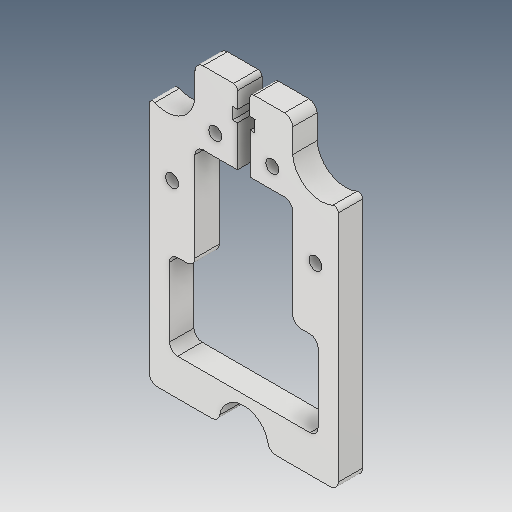
# Autodesk Inventor part: Hotend Slide Part 2
Saved by Autodesk Inventor 2017 (Build 210142000, 142)
## iProperties
Created: 2016-06-24
Part Number: Hotend Slide Part 2
Material: Acetal Resin, White
Document SubType Name: Modeling
Designer: joshm
Density: 1.425 g/cm^3
Appearance: Smooth - White
Mass: 13.5596 g
Surface Area: 60.0881 cm^2
Volume: 9.51552 cm^3
Author: joshm
Autodesk Inventor part; units mm, degrees
ref_plane "YZ Plane" through (0, 0, 0) normal (1, 0, 0) x (0, 1, 0)
ref_plane "XZ Plane" through (0, 0, 0) normal (0, 1, 0) x (-1, 0, 0)
ref_plane "XY Plane" through (0, 0, 0) normal (0, 0, 1) x (1, 0, 0)
sketch "Sketch1" plane through (0, 0, 0) normal (0, 0, 1) x (1, 0, 0)
  line L0 (-11.9794, 21.8002) -> (-11.9794, -0.1998)
  line L1 (-13.9794, -2.1998) -> (-16.2294, -2.1998)
  line L2 (12.0206, -0.1998) -> (12.0206, 21.8002)
  line L3 (16.2706, -2.1998) -> (14.0206, -2.1998)
  line L4 (-23.2294, -2.1998) -> (-23.2294, 27.0455)
  line L5 (23.2706, -2.1998) -> (23.2706, 27.0455)
  line L6 (-1.5294, 33.8002) -> (-2.7294, 33.8002)
  line L7 (1.5706, 33.8002) -> (2.7706, 33.8002)
  arc A0 (12.0206, 33.8002) -> (21.8617, 27.958) centre (18.9993, 34.346) ccw
  arc A1 (-21.8205, 27.958) -> (-11.9794, 33.8002) centre (-18.9581, 34.346) ccw
  line L8 (-1.5294, 23.8002) -> (-1.5294, 33.8002)
  line L9 (1.5706, 23.8002) -> (1.5706, 33.8002)
  circle A2 centre (17.6456, 13.5013) radius 1.6
  circle A3 centre (-17.6044, 13.5013) radius 1.6
  circle A4 centre (7.0206, 28.8002) radius 1.6
  circle A5 centre (-6.9794, 28.8002) radius 1.6
  line L10 (-1.5294, 33.8002) -> (-2.7294, 33.8002)
  line L11 (2.7706, 33.8002) -> (2.7706, 36.7002)
  line L12 (-2.7294, 36.7002) -> (-2.7294, 33.8002)
  line L13 (-2.4794, 41.7002) -> (-9.9794, 41.7002)
  line L14 (-11.9794, 39.7002) -> (-11.9794, 33.8002)
  line L15 (12.0206, 33.8002) -> (12.0206, 39.7002)
  line L16 (10.0206, 41.7002) -> (2.5206, 41.7002)
  line L17 (1.5206, 36.7002) -> (1.5206, 40.7002)
  line L18 (-1.4794, 40.7002) -> (-1.4794, 36.7002)
  arc A6 (-9.9794, 23.8002) -> (-11.9794, 21.8002) centre (-9.9794, 21.8002) ccw
  arc A7 (12.0206, 21.8002) -> (10.0206, 23.8002) centre (10.0206, 21.8002) ccw
  arc A8 (12.0206, -0.1998) -> (14.0206, -2.1998) centre (14.0206, -0.1998) ccw
  arc A9 (-13.9794, -2.1998) -> (-11.9794, -0.1998) centre (-13.9794, -0.1998) ccw
  arc A10 (12.0206, 39.7002) -> (10.0206, 41.7002) centre (10.0206, 39.7002) ccw
  arc A11 (-9.9794, 41.7002) -> (-11.9794, 39.7002) centre (-9.9794, 39.7002) ccw
  arc A12 (-1.4794, 40.7002) -> (-2.4794, 41.7002) centre (-2.4794, 40.7002) ccw
  arc A13 (2.5206, 41.7002) -> (1.5206, 40.7002) centre (2.5206, 40.7002) ccw
  arc A14 (23.2706, 27.0455) -> (21.8617, 27.958) centre (22.2706, 27.0455) ccw
  arc A15 (-21.8205, 27.958) -> (-23.2294, 27.0455) centre (-22.2294, 27.0455) ccw
  line L19 (-23.2294, -2.1998) -> (-23.2294, -30.1998)
  line L20 (-21.2294, -32.1998) -> (21.2706, -32.1998)
  line L21 (23.2706, -30.1998) -> (23.2706, -2.1998)
  line L22 (-18.2294, -4.1998) -> (-18.2294, -21.1998)
  line L23 (18.2706, -4.1998) -> (18.2706, -21.1998)
  line L24 (16.2706, -23.1998) -> (-16.2294, -23.1998)
  arc A16 (-18.2294, -21.1998) -> (-16.2294, -23.1998) centre (-16.2294, -21.1998) ccw
  arc A17 (16.2706, -23.1998) -> (18.2706, -21.1998) centre (16.2706, -21.1998) ccw
  arc A18 (18.2706, -4.1998) -> (16.2706, -2.1998) centre (16.2706, -4.1998) ccw
  arc A19 (-16.2294, -2.1998) -> (-18.2294, -4.1998) centre (-16.2294, -4.1998) ccw
  arc A20 (21.2706, -32.1998) -> (23.2706, -30.1998) centre (21.2706, -30.1998) ccw
  arc A21 (-23.2294, -30.1998) -> (-21.2294, -32.1998) centre (-21.2294, -30.1998) ccw
  line L25 (10.0206, 23.8002) -> (1.5706, 23.8002)
  line L26 (-1.5294, 23.8002) -> (-9.9794, 23.8002)
  line L27 (-2.7294, 33.8002) -> (-1.5294, 33.8002)
  line L28 (1.5706, 33.8002) -> (2.7706, 33.8002)
  line L29 (2.7706, 36.7002) -> (1.5206, 36.7002)
  line L30 (-1.4794, 36.7002) -> (-2.7294, 36.7002)
  point P0 (0, 0)
  point P1 (0, 0)
  point P2 (-23.2294, 28.8002)
  point P3 (23.2706, 28.8002)
  point P4 (-23.2294, -32.1998)
  point P5 (-18.2294, -23.1998)
  dimension "d0" = 31
  dimension "d1" = 7
  dimension "d2" = 7
  dimension "d6" = 2
  dimension "d8" = 30
  dimension "d13" = 2
  constraints: 62 end point, 38 point on circle, 34 tangent, 22 centre point, 13 equal radius, 9 perpendicular, 8 point on line, 6 parallel, 4 vertical, 3 horizontal
  measures "d0" distance of L4.start point (-23.229, 28.8)
  measures "d1" radius of A0
  measures "d2" radius of A1
  measures "d6" radius of A6
  measures "d8" distance of L4.start point (-23.229, -32.2)
  measures "d13" radius of A16
extrude "Extrusion1" add sketch "Sketch1" along normal blind 6
sketch "Sketch2" plane through (0, 0, 6) normal (0, 0, 1) x (1, 0, 0)
  line L0 (-21.2294, -32.1998) -> (21.2706, -32.1998) projected
  line L1 (0.0206, -32.1998) -> (0.0206, -28.1998)
  line L2 (0.0206, -28.1998) -> (0.0206, -34.998)
  line L3 (0.0206, -34.998) -> (0.0206, -28.1998)
  circle A0 centre (0.0206, -31.5989) radius 5.0514
  circle A1 centre (0.0206, -31.5989) radius 6.0346
  point P0 (0, 0)
  dimension "d16" = 4
  constraints: 6 end point, 2 centre point, 2 midpoint, 1 coincident, 1 collinear, 1 point on line, 1 vertical
  measures "d16" distance of L1.start L1.end
extrude "Extrusion2" cut sketch "Sketch2" against normal blind 6
fillet "Fillet1" radius 2 2 edges at (-5.984, -32.1998, 3) (6.0253, -32.1998, 3)
body "Solid1"
